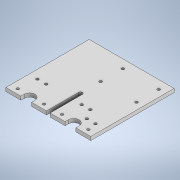
# Autodesk Inventor part: Battery Base Plate
Saved by Autodesk Inventor 2021 (Build 250183000, 183)
## iProperties
Created: 2020-07-28
Part Number: Battery Base Plate
Material: Generic
Document SubType Name: Modeling
Designer: jgray
Density: 1 g/cm^3
Appearance: Default
Author: jgray
Autodesk Inventor part; units mm, degrees
ref_plane "YZ Plane" through (0, 0, 0) normal (1, 0, 0) x (0, 1, 0)
ref_plane "XZ Plane" through (0, 0, 0) normal (0, 1, 0) x (-1, 0, 0)
ref_plane "XY Plane" through (0, 0, 0) normal (0, 0, 1) x (1, 0, 0)
sketch "Sketch1" plane through (0, 0, 0) normal (0, 1, 0) x (-1, 0, 0)
  line L0 (0, 0) -> (118.5, 0)
  line L1 (118.5, 0) -> (118.5, -116.2)
  line L2 (118.5, -116.2) -> (0, -116.2)
  line L3 (0, -116.2) -> (0, 0)
  dimension "d0" = 118.5
  dimension "d1" = 116.2
  constraints: 8 end point, 2 parallel, 1 horizontal, 1 perpendicular
  measures "d0" distance of L1.end L2.end
  measures "d1" distance of L0.end L1.end
extrude "Extrusion1" add sketch "Sketch1" along normal blind 5
sketch "Sketch2" plane through (0, 5, 0) normal (0, 1, 0) x (1, 0, 0)
  line L0 (-59.5, 73.2) -> (-9.5, 73.2)
  line L1 (-9.5, 73.2) -> (-9.5, 104.2)
  line L2 (-9.5, 104.2) -> (-59.5, 104.2)
  line L3 (-59.5, 104.2) -> (-59.5, 73.2)
  line L4 (0, 116.2) -> (-118.5, 116.2) projected
  line L5 (-118.5, 116.2) -> (-118.5, 0) projected
  point P0 (0, 0)
  dimension "d4" = 12
  dimension "d5" = 31
  dimension "d6" = 50
  dimension "d7" = 59
  constraints: 8 end point, 4 coincident, 2 parallel, 1 horizontal, 1 perpendicular
  measures "d4" distance between parallel lines of L4 L2
  measures "d5" distance between parallel lines of L2 L0
  measures "d6" distance between parallel lines of L1 L3
  measures "d7" distance between parallel lines of L5 L3
hole "Hole1" at (-59.5, 5, -73.2) at (-9.5, 5, -73.2) at (-59.5, 5, -104.2) at (-9.5, 5, -104.2) direction (0, -1, 0) diameter 3.8 end through all
sketch "Sketch3" plane through (0, 5, 0) normal (0, 1, 0) x (1, 0, 0)
  line L0 (-59.25, -19.9196) -> (-59.25, 121.041) construction
  line L1 (-118.5, 0) -> (0, 0) projected
  line L2 (-61.775, 0) -> (-56.725, 0)
  line L3 (-56.725, 0) -> (-56.725, 45)
  line L4 (-61.775, 45) -> (-61.775, 0)
  arc A0 (-56.725, 45) -> (-61.775, 45) centre (-59.25, 45) ccw
  point P0 (-59.25, 0)
  dimension "d18" = 5.05
  dimension "d19" = 45
  constraints: 8 end point, 3 point on line, 2 point on circle, 1 centre point, 1 horizontal, 1 midpoint, 1 parallel, 1 perpendicular, 1 vertical, 1 other
  measures "d18" distance between parallel lines of L3 L4
  measures "d19" distance of L2.end L3.end
extrude "Extrusion2" cut sketch "Sketch3" against normal blind 10
sketch "Sketch4" plane through (0, 5, 0) normal (0, 1, 0) x (1, 0, 0)
  line L0 (-148.0192, 32) -> (31.7399, 32) construction
  line L1 (-56.725, 0) -> (0, 0) construction
  line L2 (-118.5, 116.2) -> (-118.5, 0) construction
  line L3 (-59.25, 61.4977) -> (-59.25, -14.0332) construction
  line L4 (-61.775, 45) -> (-61.775, 0) construction
  arc A0 (-56.725, 45) -> (-61.775, 45) centre (-59.25, 45) ccw construction
  line L5 (-27.032, 18.5) -> (18.1948, 18.5) construction
  line L6 (0, 0) -> (0, 116.2) construction
  point P0 (-106.5, 32)
  point P1 (-94.5, 32)
  point P2 (-44.75, 32)
  point P3 (-32.75, 32)
  point P4 (-59.25, 47.525)
  point P5 (-12, 18.5)
  point P6 (-24, 18.5)
  dimension "d22" = 32
  dimension "d23" = 12
  dimension "d24" = 12
  dimension "d25" = 12
  dimension "d26" = 14.5
  dimension "d27" = 18.5
  dimension "d28" = 12
  dimension "d29" = 12
  constraints: 7 point on line, 6 end point, 2 horizontal, 1 parallel, 1 point on circle
  measures "d22" distance between parallel lines of L1 L0
  measures "d23" distance of point (-94.5, 32) point (-106.5, 32)
  measures "d24" distance of point (-32.75, 32) point (-44.75, 32)
  measures "d25" distance from line of point (-106.5, 32) L2
  measures "d26" distance from line of point (-44.75, 32) L3
  measures "d27" distance between parallel lines of L1 L5
  measures "d28" distance from line of L6 point (-12, 18.5)
  measures "d29" distance of point (-12, 18.5) point (-24, 18.5)
hole "Hole2" at (-106.5, 5, -32) at (-94.5, 5, -32) at (-44.75, 5, -32) at (-32.75, 5, -32) at (-12, 5, -18.5) at (-24, 5, -18.5) direction (0, -1, 0) diameter 3.8 end through all
sketch "Sketch5" plane through (0, 5, 0) normal (0, 1, 0) x (1, 0, 0)
  line L0 (-134.8767, 6.5) -> (26.057, 6.5) construction
  line L1 (-56.725, 0) -> (0, 0) construction
  line L2 (0, 0) -> (0, 116.2) construction
  line L3 (-118.5, 116.2) -> (-118.5, 0) construction
  line L4 (-59.25, 58.1) -> (-59.25, -13.4303) construction
  arc A0 (-56.725, 45) -> (-61.775, 45) centre (-59.25, 45) ccw construction
  point P0 (-108.5, 6.5)
  point P1 (-71.75, 6.5)
  point P2 (-46.75, 6.5)
  point P3 (-10, 6.5)
  point P4 (-59.25, 47.525)
  dimension "d37" = 6.5
  dimension "d38" = 10
  dimension "d39" = 10
  dimension "d40" = 12.5
  dimension "d41" = 12.5
  constraints: 5 point on line, 4 end point, 1 horizontal, 1 point on circle, 1 vertical
  measures "d37" distance between parallel lines of L1 L0
  measures "d38" distance from line of L2 point (-10, 6.5)
  measures "d39" distance from line of L3 point (-108.5, 6.5)
  measures "d40" distance from line of point (-71.75, 6.5) L4
  measures "d41" distance from line of point (-46.75, 6.5) L4
hole "Hole3" at (-108.5, 5, -6.5) at (-71.75, 5, -6.5) at (-46.75, 5, -6.5) at (-10, 5, -6.5) direction (0, -1, 0) diameter 3.8 end through all
sketch "Sketch6" plane through (0, 5, 0) normal (0, 1, 0) x (1, 0, 0)
  line L0 (-90.1375, 21.1453) -> (-90.1375, -29.1073) construction
  line L1 (-28.4418, 11.0948) -> (-28.4418, -20.2874) construction
  line L2 (-90.1375, -5.5) -> (-90.1375, 4.5) construction
  line L3 (-82.6375, -5.5) -> (-82.6375, 4.5)
  line L4 (-97.6375, 4.5) -> (-97.6375, -5.5)
  arc A0 (-97.6375, -5.5) -> (-82.6375, -5.5) centre (-90.1375, -5.5) ccw
  arc A1 (-82.6375, 4.5) -> (-97.6375, 4.5) centre (-90.1375, 4.5) ccw
  line L5 (-28.4418, -5.5) -> (-28.4418, 4.5) construction
  line L6 (-20.9418, -5.5) -> (-20.9418, 4.5)
  line L7 (-35.9418, 4.5) -> (-35.9418, -5.5)
  arc A2 (-35.9418, -5.5) -> (-20.9418, -5.5) centre (-28.4418, -5.5) ccw
  arc A3 (-20.9418, 4.5) -> (-35.9418, 4.5) centre (-28.4418, 4.5) ccw
  line L8 (-56.725, 0) -> (0, 0) projected
  line L9 (-118.5, 0) -> (-61.775, 0) projected
  line L10 (-118.5, 0) -> (-61.775, 0) projected
  line L11 (-97.6375, 0) -> (-82.6375, 0)
  line L12 (-35.9418, 0) -> (-20.9418, 0)
  point P0 (-90.1375, -0.5)
  point P1 (-28.4418, -0.5)
  point P2 (-97.6375, 0)
  point P3 (-82.6375, 0)
  dimension "d49" = 15
  dimension "d50" = 15
  dimension "d51" = 4.5
  dimension "d52" = 4.5
  dimension "d53" = 10
  dimension "d54" = 10
  constraints: 24 end point, 12 point on line, 8 point on circle, 8 tangent, 4 centre point, 2 midpoint, 2 parallel, 2 vertical
  measures "d49" diameter of A1
  measures "d50" diameter of A3
  measures "d51" distance from line of L8 L5.end
  measures "d52" distance from line of L9 L2.end
  measures "d53" distance of L2.start L2.end
  measures "d54" distance of L5.start L5.end
extrude "Extrusion3" cut sketch "Sketch6" against normal through all contours L9 L4 A1 L3 | L8 L7 A3 L6
body "Solid1"
